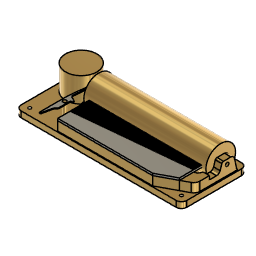
Sankyo SZ72S 72-note Movement (Autodesk Fusion 360 design; units mm, degrees)
Autodesk Fusion 360 part; units mm, degrees
note: some values were not read from the file. Set by a fixed rule: the direction of a hole.
sketch "Sketch1" plane through (0, 0, 0) normal (0, 0, 1) x (1, 0, 0)
  line L0 (-2, 67) -> (176, 67)
  line L1 (182, 61) -> (182, -2)
  line L2 (176, -8) -> (-2, -8)
  line L3 (-8, -2) -> (-8, 61)
  arc A0 (-2, 67) -> (-8, 61) centre (-2, 61) ccw
  arc A1 (-8, -2) -> (-2, -8) centre (-2, -2) ccw
  arc A2 (176, -8) -> (182, -2) centre (176, -2) ccw
  arc A3 (182, 61) -> (176, 67) centre (176, 61) ccw
  circle A4 centre (13, 46) radius 18
  line L4 (13, 46) -> (182, 46) construction
  line L5 (26.5, 17.7353) -> (26.5, -15.65)
  line L6 (26.5, -15.65) -> (27.792, -15.65)
  line L7 (27.792, -15.65) -> (30.4775, -3.0154)
  line L8 (30.4775, -3.0154) -> (33.1331, -0.3598)
  line L9 (33.1331, -0.3598) -> (33.1331, 12.6339)
  arc A5 (34.4528, 13.9535) -> (33.1331, 12.6339) centre (34.4528, 12.6339) ccw
  line L10 (34.4528, 13.9535) -> (35.5, 13.9535)
  line L11 (35.5, 13.9535) -> (35.5, 15.5)
  line L12 (35.5, 15.5) -> (30.233, 18.1468)
  arc A6 (28.8117, 20.7748) -> (30.233, 18.1468) centre (31.4049, 20.4789) ccw
  line L13 (28.8117, 20.7748) -> (30.233, 37.184)
  arc A7 (30.6827, 38.1755) -> (30.233, 37.184) centre (31.8618, 37.0429) ccw
  line L14 (30.6827, 38.1755) -> (30.8526, 40.1364)
  line L15 (30.8526, 40.1364) -> (30.7728, 40.1433)
  arc A8 (30.7728, 40.1433) -> (28.8937, 38.602) centre (30.6227, 38.4103) ccw
  line L16 (28.8937, 38.602) -> (26.9786, 21.3337)
  line L17 (26.9786, 21.3337) -> (26.5238, 17.8005)
  line L18 (26.5238, 17.8005) -> (26.5, 17.7353)
  line L19 (256.8449, 63.9308) -> (263.6449, 63.9308)
  line L20 (263.6449, 63.9308) -> (263.6449, -11.0692)
  line L21 (263.6449, -11.0692) -> (256.8449, -11.0692)
  line L22 (256.8449, -11.0692) -> (256.8449, 63.9308)
  circle A9 centre (245.6449, 41.8769) radius 17
  line L23 (244.2449, -10.0692) -> (246.6449, -10.0692)
  line L24 (246.6449, -10.0692) -> (246.6449, 16.9308)
  line L25 (246.6449, 16.9308) -> (244.2449, 16.9308)
  line L26 (244.2449, 16.9308) -> (244.2449, -10.0692)
  line L27 (39, 7.3298) -> (39, -7)
  line L28 (39, -7) -> (148, -7)
  line L29 (148, -7) -> (168, 3.6342)
  line L30 (168, 3.6342) -> (168, 20)
  line L31 (168, 20) -> (39, 7.3298)
  line L32 (40, 7.428) -> (40, 33)
  line L33 (39, 33) -> (39, 7.3298)
  line L34 (39, 33) -> (40, 33)
  line L35 (168, 3.6342) -> (176.8389, 8.3339)
  arc A10 (176.8389, 8.3339) -> (180.5526, 14.5146) centre (173.5526, 14.5146) ccw
  line L36 (180.5526, 14.5146) -> (180.5526, 58)
  line L37 (180.5526, 58) -> (173.0526, 58)
  line L38 (173.0526, 58) -> (173.0526, 25.5732)
  arc A11 (168, 20) -> (173.0526, 25.5732) centre (167.4526, 25.5732) ccw
  line L39 (30.8526, 63.2333) -> (33, 63.2333)
  line L40 (33, 63.2333) -> (33, 29)
  line L41 (33, 29) -> (30.8526, 29)
  line L42 (30.8526, 29) -> (30.8526, 63.2333)
  circle A12 centre (30, 10) radius 2
  point P0 (182, 67)
  point P1 (182, -8)
  point P2 (-8, -8)
  point P3 (174, 0)
  point P4 (87, 62)
  point P5 (245.6449, 41.8769)
  dimension "d7" = 6
  dimension "d9" = 46
  dimension "d10" = 74
  dimension "d12" = 16
  dimension "d13" = 46
  dimension "d14" = 36
  dimension "d15" = 13.5
  dimension "d16" = 13
  dimension "d17" = 7.65
  dimension "d19" = 161
  dimension "d20" = 21
  dimension "d21" = 54
  dimension "d22" = 21
  dimension "d23" = 169
  dimension "d25" = 12
  dimension "d30" = 75
  dimension "d31" = 6.8
  dimension "d32" = 18
  dimension "cylinder_diameter" = 34
  dimension "comb_thickness" = 2.4
  dimension "comb_VOffset" = 17
  dimension "comb_HOffset" = 1
  dimension "d38" = 1
  dimension "comb_tineWidth" = 1
  dimension "comb_width" = 129
  dimension "d58" = 40
  dimension "d59" = 5.61
  dimension "d60" = 27
  dimension "d61" = 152
  dimension "d62" = 109
  dimension "d63" = 7.5
  dimension "d64" = 39
  dimension "d65" = 7
  dimension "d66" = 5.6
  dimension "d67" = 58
  dimension "d107" = 10
  dimension "d108" = 30
  dimension "d109" = 4
  constraint horizontal L0
  constraint vertical L1
  constraint horizontal L2
  constraint vertical L3
  constraint tangent L0 A0
  constraint tangent L3 A0
  constraint coincident P2 L2
  constraint coincident P2 L3
  constraint tangent L2 A1
  constraint tangent L3 A1
  constraint equal A0 A1
  constraint coincident P1 L1
  constraint coincident P1 L2
  constraint tangent L1 A2
  constraint tangent L2 A2
  constraint equal A0 A2
  constraint coincident P0 L0
  constraint coincident P0 L1
  constraint tangent L0 A3
  constraint tangent L1 A3
  constraint equal A0 A3
  constraint perpendicular L1 L4
  constraint coincident L1 L4.end
  constraint perpendicular L2 L5
  constraint perpendicular L5 L6
  constraint perpendicular L2 L9
  constraint tangent L9 A5
  constraint tangent A5 L10
  constraint perpendicular L9 L10
  constraint perpendicular L10 L11
  constraint tangent L12 A6
  constraint tangent L13 A7
  constraint parallel L13 L14
  constraint perpendicular L14 L15
  constraint tangent L15 A8
  constraint tangent A8 L16
  constraint coincident A4.centre L4.start
  constraint horizontal L19
  constraint vertical L20
  constraint horizontal L21
  constraint vertical L22
  constraint coincident P5 A9.centre
  constraint horizontal L23
  constraint vertical L24
  constraint horizontal L25
  constraint vertical L26
  constraint perpendicular L2 L27
  constraint perpendicular L27 L28
  constraint perpendicular L28 L30
  constraint vertical L32
  constraint vertical L33
  constraint coincident L31 L32.start
  constraint perpendicular L32 L34
  constraint parallel L29 L35
  constraint tangent L35 A10
  constraint perpendicular L1 L37
  constraint tangent L38 A11
  constraint tangent A10 L36
  constraint tangent L31 A11
  constraint vertical L38
  constraint vertical L36
  constraint horizontal L39
  constraint vertical L40
  constraint horizontal L41
  constraint vertical L42
  measures "d7" radius of A0
  measures "d9" vertical distance of origin A4.centre
  measures "d10" horizontal distance of A4.centre P4
  measures "d12" distance of P4 L4
  measures "d13" distance of P3 L4
  measures "d14" diameter of A4
  measures "d15" distance of A4.centre L5
  measures "d16" horizontal distance of origin A4.centre
  measures "d17" distance of L2 L6
  measures "d19" horizontal distance of A4.centre P3
  measures "d20" distance of L3 A4.centre
  measures "d21" distance of L2 L4
  measures "d22" distance of L0 L4
  measures "d23" distance of L1 A4.centre
  measures "d25" angle of L5 L7
  measures "d30" distance of L19.end L20.end
  measures "d31" distance of L20.end L21.end
  measures "d32" distance of L20 P5
  measures "cylinder_diameter" diameter of A9
  measures "comb_thickness" distance of L23.start L23.end
  measures "comb_VOffset" distance of L20 L24
  measures "comb_HOffset" distance of L21 L23
  measures "d38" distance of L2 L28
  measures "comb_tineWidth" distance of L32.end L33.start
  measures "comb_width" distance of L27 L30
  measures "d58" distance of L27.end L33.start
  measures "d59" angle of L28 L31
  measures "d60" distance of L28 L30.end
  measures "d61" angle of L28 L29
  measures "d62" distance of L27.end L28.end
  measures "d63" distance of L36.end L37.end
  measures "d64" distance of origin L27
  measures "d65" radius of A10
  measures "d66" radius of A11
  measures "d67" distance of P3 L37
  measures "d107" vertical distance of origin A12.centre
  measures "d108" horizontal distance of origin A12.centre
  measures "d109" diameter of A12
extrude "Extrude1" add sketch "Sketch1" along normal blind 6.8 contours L0 L1 L2 L3 A0 A1 A2 A3 A4 L5 L7 L8 L9 A5 L10 L11 L12 A6 L13 A7 L14 L16 L17 L18 L39 L40 L41 L42 | L2 A4 L5 L7 L8 L9 A5 L10 L11 L12 A6 L13 A7 L14 L15 A8 L16 L17 L18 | A4 A8 L16 L42 | A4 L39 L40 L41 L42 | A4 L42 | A4 L15 A8 L42 | L27 L28 L29 L30 L31 | L31 L32 L33 L34 | L30 L35 A10 L36 L37 L38 A11 | A12 makes body 1
extrude "Extrude2" add sketch "Sketch1" along normal blind 35 contours A4 A8 L16 | A4 A8 L16 L42 | A4 L42 bodies 1
extrude "Extrude3" add sketch "Sketch1" along normal blind 2.4 from surface at 17 separate body contours L27 L28 L29 L30 L31 makes body 2
extrude "Extrude4" add sketch "Sketch1" along normal blind 2.4 from surface at 17 contours L31 L32 L33 L34 bodies 2
pattern_linear "R-Pattern1" count 72 spacing 1.8028 along (1, 0, 0) of "Extrude4"
copy_body "Body->Comp2" bodies 1 removing the originals makes body 3 in component "Base"
copy_body "Body->Comp1" bodies 2 removing the originals makes body 4 in component "Comb"
extrude "Extrude1'" add sketch "Sketch1" along normal blind 17 contours A4 L39 L40 L41 L42 | L27 L28 L29 L30 L31 | L30 L35 A10 L36 L37 L38 A11 bodies 3 in component "Base"
sketch "Sketch2" plane through (180.5526, 0, 0) normal (1, 0, 0) x (0, 1, 0)
  line L0 (56.666, 8.7988) -> (54.1843, 20.0608)
  arc A0 (54.1843, 20.0608) -> (50.278, 23.2) centre (50.278, 19.2) ccw
  line L1 (50.278, 23.2) -> (41.722, 23.2)
  arc A1 (41.722, 23.2) -> (39.8216, 21.8233) centre (41.722, 21.2) ccw
  line L2 (39.8216, 21.8233) -> (37.8307, 15.7538)
  arc A2 (33.7531, 12.8) -> (37.8307, 15.7538) centre (33.7531, 17.0913) ccw
  line L3 (33.7531, 12.8) -> (33.7531, 6.8)
  line L4 (33.7531, 6.8) -> (59.1531, 6.8)
  arc A3 (56.666, 8.7988) -> (59.1531, 6.8) centre (59.1531, 9.3468) ccw
  line L5 (14.5146, 6.8) -> (58, 6.8)
  line L6 (58, 6.8) -> (58, 17)
  line L7 (58, 17) -> (14.5146, 17)
  line L8 (14.5146, 17) -> (14.5146, 6.8)
  line L9 (33.7531, 12.8) -> (55.7843, 12.8) construction
  circle A4 centre (46, 18) radius 2
  line L10 (46, 18) -> (46, 0) construction
  line L11 (58, 6.8) -> (25.5732, 6.8)
  line L12 (25.5732, 6.8) -> (25.5732, 17)
  line L13 (25.5732, 17) -> (58, 17)
  line L14 (58, 17) -> (58, 6.8)
  line L15 (33.7531, 12.8) -> (25.5732, 12.8)
  line L16 (46, 18) -> (46, 23.2) construction
  line L17 (29, 6.8) -> (63.2333, 6.8)
  line L18 (63.2333, 6.8) -> (63.2333, 17)
  line L19 (63.2333, 17) -> (29, 17)
  line L20 (29, 17) -> (29, 6.8)
  point P0 (46, 0)
  dimension "d76" = 2
  dimension "d77" = 4
  dimension "d78" = 16.4
  dimension "d79" = 4.2913
  dimension "d81" = 25.4
  dimension "d82" = 71.84
  dimension "d83" = 77.573
  dimension "d84" = 2.5468
  dimension "d85" = 6
  dimension "d86" = 18
  dimension "d87" = 4
  constraint tangent L0 A0
  constraint tangent L1 A1
  constraint tangent L2 A2
  constraint perpendicular L1 L3
  constraint perpendicular L3 L4
  constraint tangent L0 A3
  constraint tangent L4 A3
  constraint tangent A0 L1
  constraint perpendicular L3 L9
  constraint tangent A2 L9
  constraint coincident L0 L9.end
  constraint coincident L4.end L5
  constraint coincident L3.end L5
  constraint coincident A4.centre L10.start
  constraint coincident P0 L10.end
  constraint vertical L10
  constraint coincident A2.start L3.start
  constraint coincident L12 L15.end
  constraint perpendicular L12 L15
  constraint coincident L1 L16.end
  constraint perpendicular L1 L16
  constraint midpoint L1 L16.end
  constraint tangent A1 L2
  measures "d76" radius of A1
  measures "d77" radius of A0
  measures "d78" distance of L1 L4
  measures "d79" radius of A2
  measures "d81" distance of L3.end L4.end
  measures "d82" angle of L2 L4
  measures "d83" angle of L0 L4
  measures "d84" radius of A3
  measures "d85" distance of L3.end A2.start
  measures "d86" distance of A4.centre P0
  measures "d87" diameter of A4
extrude "Extrude2'" cut sketch "Sketch2" against normal up to surface (149.7 mm away) contours L0 A3 L6 L7 L13 L14 L19 | A3 L6 L14 L17 L18 L19 | L7 A4 L13 L19 | L2 A2 L7 L13 L15 L19 L20 | L7 L12 L13 L15 L20 picked at (45.4904, 16.7623) bodies 3 in component "Base"
extrude "Extrude3'" add sketch "Sketch2" against normal up to surface (7.5 mm away) contours L0 A0 L1 A1 L2 L7 A4 L13 L19 bodies 3 in component "Base"
extrude "Extrude4'" add sketch "Sketch2" against normal up to surface (2.1474 mm away) from surface at -147.5526 contours L0 A0 L1 A1 L2 L7 A4 L13 L19 bodies 3 in component "Base"
sketch "Sketch1 (2)" plane through (0, 0, 0) normal (1, 0, 0) x (0, 0, -1) in component "Cylinder"
  circle A0 centre (0, 0) radius 17
  circle A1 centre (0, 0) radius 2
  dimension "d95" = 34
  dimension "d96" = 4
  constraint coincident A0.centre A1.centre
  measures "d95" diameter of A0
  measures "d96" diameter of A1
extrude "Extrude1''" add sketch "Sketch1 (2)" along normal up to surface (140.0526 mm away) from surface at 33 separate body makes body 5 in component "Cylinder"
extrude "Extrude1'''" add sketch "Sketch1" along normal blind 1 from surface at 22.5 separate body contours L2 A4 L5 L7 L8 L9 A5 L10 L11 L12 A6 L13 A7 L14 L15 A8 L16 L17 L18 | L2 L5 L6 L7 | A4 A8 L16 makes body 6 in component "Switch"
extrude "Extrude5" add sketch "Sketch1" along normal blind 23.5 contours A12 bodies 3 in component "Base"
hole "Hole1" at (0, 0, 0) at (87, 62, 0) at (174, 0, 0) direction (0, 0, 1) diameter 3.332 end up to surface (6.8 mm away) bodies 3 in component "Base"
thread "Thread1" "ISO Metric profile 4.0 M4x0.7 6H" thread offset 0 thread depth 10 in component "Base"
component "Base" placed x (1, 0, 0) y (0, 1, 0) z (0, 0, 1) at (0, 0, 0)
component "Comb" placed x (1, 0, 0) y (0, 1, 0) z (0, 0, 1) at (0, 0, 0)
component "Cylinder" placed x (1, 0, 0) y (0, 1, 0) z (0, 0, 1) at (0, 46, 18)
component "Switch" placed x (1, 0, 0) y (0, 1, 0) z (0, 0, 1) at (0, 0, 0)
equation "width = 190 mm"
equation "depth = 75 mm"
equation "base_thickness = 6.8 mm"
equation "d26 = base_thickness"
equation "d30 = depth"
equation "d31 = base_thickness"
equation "d38 = comb_HOffset"
equation "d40 = comb_VOffset"
equation "d41 = comb_thickness"
equation "d43 = comb_VOffset"
equation "d44 = comb_thickness"
equation "d49 = comb_width - comb_tineWidth"
equation "switch_VOffset = 22.5 mm"
equation "switch_thickness = 1 mm"
equation "cylinder_VOffset = 18 mm"
equation "key_length = 16.3 mm"
equation "key_width = 38 mm"
equation "key_shaftDiameter = 4 mm"
equation "key_shaftLength = 11.25 mm"
equation "d70 = comb_VOffset"
equation "d86 = cylinder_VOffset"
equation "d95 = cylinder_diameter"
equation "d104 = switch_VOffset"
equation "d105 = switch_thickness"
equation "d110 = switch_VOffset + switch_thickness"
